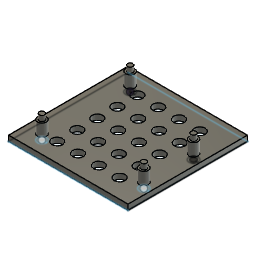
Sumobot Lattice v2 (Autodesk Fusion 360 design; units mm, degrees)
Autodesk Fusion 360 part; units mm, degrees
sketch "Sketch1" plane through (0, 0, 0) normal (0, 1, 0) x (1, 0, 0)
  circle A0 centre (0, 0) radius 1.5
  circle A1 centre (50.8, -15.2) radius 1.5
  circle A2 centre (50.8, -43.1) radius 1.5
  circle A3 centre (-1.3, -48.2) radius 1.5
  line L0 (-10, 8.8) -> (57, 8.8)
  line L1 (57, 8.8) -> (57, -58.2)
  line L2 (57, -58.2) -> (-10, -58.2)
  line L3 (-10, -58.2) -> (-10, 8.8)
  circle A4 centre (50.8, -15.2) radius 2.5
  circle A5 centre (50.8, -43.1) radius 2.5
  circle A6 centre (-1.3, -48.2) radius 2.5
  circle A7 centre (0, 0) radius 2.5
  dimension "d1" = 3
  dimension "d2" = 3
  dimension "d3" = 50.8
  dimension "d4" = 15.2
  dimension "d5" = 3
  dimension "d6" = 27.9
  dimension "d7" = 3
  dimension "d8" = 5.1
  dimension "d9" = 1.3
  dimension "d10" = 67
  dimension "d11" = 67
  dimension "d12" = 10
  dimension "d13" = 10
  dimension "d16" = 5
  dimension "d17" = 5
  dimension "d18" = 5
  dimension "d19" = 5
  constraint coincident A0.centre A7.centre
  constraint horizontal L0
  constraint vertical L1
  constraint horizontal L2
  constraint vertical L3
  constraint concentric A1 A4
  constraint concentric A2 A5
  constraint concentric A3 A6
  constraint concentric A0 A7
  measures "d1" diameter of A0
  measures "d2" diameter of A1
  measures "d3" horizontal distance of A0.centre A1.centre
  measures "d4" vertical distance of A0.centre A1.centre
  measures "d5" diameter of A2
  measures "d6" distance of A1.centre A2.centre
  measures "d7" diameter of A3
  measures "d8" vertical distance of A2.centre A3.centre
  measures "d9" horizontal distance of A0.centre A3.centre
  measures "d10" distance of L0.start L0.end
  measures "d11" distance of L0.start L2.end
  measures "d12" distance of A0.centre L3
  measures "d13" distance of A3.centre L2
  measures "d16" diameter of A4
  measures "d17" diameter of A5
  measures "d18" diameter of A6
  measures "d19" diameter of A7
extrude "Extrude1" add sketch "Sketch1" along normal blind 13 contours A0 | A1 | A2 | A3 makes body 1 at (51.2777, 8.6667, 13.7781) makes body 2 at (52.0799, 8.6667, 42.3178) makes body 3 at (1.4925, 8.6667, 0.1494) makes body 4 at (-2.6822, 8.6667, 48.7827)
extrude "Extrude3" add sketch "Sketch1" along normal blind 10 contours A5 bodies 2
extrude "Extrude4" add sketch "Sketch1" along normal blind 10 contours A4 bodies 1
extrude "Extrude5" add sketch "Sketch1" along normal blind 10 contours A6 bodies 4
extrude "Extrude6" add sketch "Sketch1" along normal blind 10 contours A7 bodies 3
extrude "Extrude7" add sketch "Sketch1" along normal blind 3 contours L0 L1 L2 L3 bodies 1 2 3 4
sketch "Sketch2" plane through (0, 3, 0) normal (0, 1, 0) x (-1, 0, 0)
  circle A0 centre (0, 0) radius 2.5
  circle A1 centre (-50.8, 15.2) radius 2.5
  circle A2 centre (1.3, 48.2) radius 2.5
  circle A3 centre (-50.8, 43.1) radius 2.5
  line L0 (10, 58.2) -> (-57, 58.2)
  line L1 (-57, 58.2) -> (-57, -8.8)
  line L2 (-57, -8.8) -> (10, -8.8)
  line L3 (10, -8.8) -> (10, 58.2)
  circle A4 centre (-6.7207, 2.6289) radius 3
  circle A5 centre (-18.3874, 2.6289) radius 3
  circle A6 centre (-30.054, 2.6289) radius 3
  circle A7 centre (-41.7207, 2.6289) radius 3
  circle A8 centre (-6.7207, 13.8789) radius 3
  circle A9 centre (-18.3874, 13.8789) radius 3
  circle A10 centre (-30.054, 13.8789) radius 3
  circle A11 centre (-41.7207, 13.8789) radius 3
  circle A12 centre (-6.7207, 25.1289) radius 3
  circle A13 centre (-18.3874, 25.1289) radius 3
  circle A14 centre (-30.054, 25.1289) radius 3
  circle A15 centre (-41.7207, 25.1289) radius 3
  circle A16 centre (-6.7207, 36.3789) radius 3
  circle A17 centre (-18.3874, 36.3789) radius 3
  circle A18 centre (-30.054, 36.3789) radius 3
  circle A19 centre (-41.7207, 36.3789) radius 3
  circle A20 centre (-6.7207, 47.6289) radius 3
  circle A21 centre (-18.3874, 47.6289) radius 3
  circle A22 centre (-30.054, 47.6289) radius 3
  circle A23 centre (-41.7207, 47.6289) radius 3
  dimension "d37" = 6
  dimension "d40" = -35
  dimension "d41" = 45
  measures "d37" diameter of A4
extrude "Extrude8" cut sketch "Sketch2" against normal blind 3 contours A4 | A5 | A6 | A7 | A8 | A9 | A10 | A11 | A12 | A13 | A14 | A15 | A16 | A17 | A18 | A19 | A20 | A21 | A22 | A23 bodies 1
extrude "Extrude2" [suppressed]
equation "d1 = HoleSize"
equation "d2 = HoleSize"
equation "d5 = HoleSize"
equation "d7 = HoleSize"
equation "HoleSize = 3 mm"
equation "PostSize = 5 mm"
equation "d16 = PostSize"
equation "d17 = PostSize"
equation "d18 = PostSize"
equation "d19 = PostSize"
equation "PostHeight = 10 mm"
equation "PegHeight = 3 mm"
equation "d22 = PostHeight + PegHeight"
equation "d24 = PostHeight"
equation "d26 = PostHeight"
equation "d28 = PostHeight"
equation "d30 = PostHeight"
equation "d32 = PostHeight"
equation "PlatformHeight = 3 mm"
equation "d35 = PlatformHeight"
equation "d42 = -PlatformHeight"
